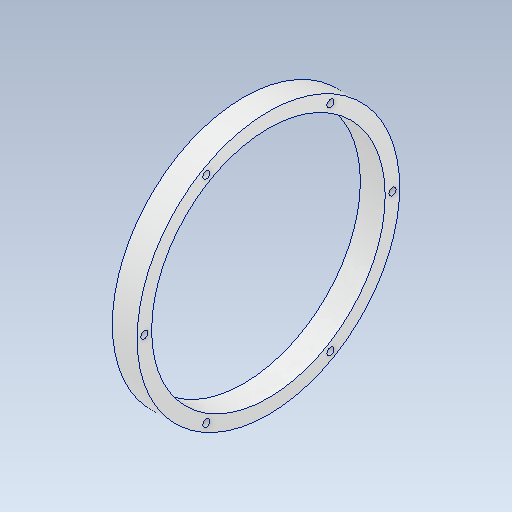
# Autodesk Inventor part: Adapter_stages_planetary
Saved by Autodesk Inventor 2021 (Build 250183000, 183)
## iProperties
Created: 2020-05-12
Part Number: Adapter_stages_planetary
Material: Aluminum 6061
Document SubType Name: Modeling
Designer: avi41
Density: 2.7 g/cm^3
Appearance: Aluminum - Flat
Mass: 177.082 g
Surface Area: 247.251 cm^2
Volume: 65.5859 cm^3
Author: avi41
Autodesk Inventor part; units mm, degrees
ref_plane "YZ Plane" through (0, 0, 0) normal (1, 0, 0) x (0, 1, 0)
ref_plane "XZ Plane" through (0, 0, 0) normal (0, 1, 0) x (-1, 0, 0)
ref_plane "XY Plane" through (0, 0, 0) normal (0, 0, 1) x (1, 0, 0)
sketch "Sketch1" plane through (0, 0, 0) normal (0, 1, 0) x (-1, 0, 0)
  line L0 (0, -83.3) -> (0, -70.7) construction
  line L1 (-10.78, 0) -> (10.78, 0) construction
  line L2 (-7.7, -72.5) -> (7.7, -72.5)
  line L3 (-7.7, -72.5) -> (-7.7, -81.5)
  line L4 (-7.7, -81.5) -> (7.7, -81.5)
  line L5 (7.7, -81.5) -> (7.7, -72.5)
  dimension "d30" = 15.4
  dimension "d31" = 9
  dimension "d47" = 72.5
  constraints: 8 end point, 3 perpendicular, 1 vertical, 1 other
  measures "d30" distance of L3.end L4.end
  measures "d31" distance between parallel lines of L2 L4
  measures "d47" distance between parallel lines of L1 L2
revolve "Revolution1" add sketch "Sketch1" angle 360 about axis through (0, 0, 0) along (-1, 0, 0)
sketch "Sketch2" plane through (-7.7, 0, 0) normal (-1, 0, 0) x (0, 0, 1)
  line L0 (0, 114.1) -> (0, -114.1) construction
  line L1 (-114.1, 0) -> (114.1, 0) construction
  circle A0 centre (0, 0) radius 72.5 projected
  circle A1 centre (0, 0) radius 81.5 projected
  circle A2 centre (0, 0) radius 77 construction
  point P0 (-77, 0)
  dimension "d33" = 4.5
  dimension "d34" = 4.5
  constraints: 1 coincident, 1 horizontal alignment, 1 point on line, 2 other
hole "Hole1" at (-7.7, 0, -77) direction (1, 0, 0) diameter 4.5 end through all clearance for "Flat Head Machine Screw" size "M4" standard "Ansi Metric M Profile"
pattern_circular "Circular Pattern1" count 6 over 360 about axis through (-10, 0, 0) along (1, 0, 0) of "Hole1"
equation "\"d33\" = d34"
equation "\"D_ring\" = D_ext"
equation "\"D_ext\" = 139.15534"
body "Solid1"
